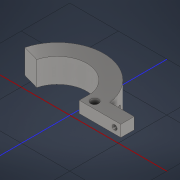
# Autodesk Inventor part: holder2_clamp
Saved by Autodesk Inventor 2021 (Build 250183000, 183)
## iProperties
Created: 2021-06-04
Part Number: holder2_clamp
Material: Steel, Mild
Document SubType Name: Modeling
Designer: Watchdog
Density: 7.85 g/cm^3
Appearance: Semi-Polished
Author: Watchdog
Autodesk Inventor part; units mm, degrees
ref_plane "YZ Plane" through (0, 0, 0) normal (1, 0, 0) x (0, 1, 0)
ref_plane "XZ Plane" through (0, 0, 0) normal (0, 1, 0) x (-1, 0, 0)
sketch "Sketch1" plane through (0, 0, 0) normal (0, 1, 0) x (-1, 0, 0)
  line L0 (5, 0) -> (16.619, -3)
  line L1 (5, 0) -> (-7, 0)
  arc A0 (-7, 0) -> (16.619, -3) centre (5, 0) ccw
  line L2 (0, 0) -> (-12, 0)
  arc A1 (-14, 0) -> (23.3548, -4.9094) centre (5, 0) ccw
  line L3 (16.619, -3) -> (23.3548, -4.9094)
  line L4 (-7, 0) -> (-14, 0)
  point P0 (-7, 0)
  dimension "d0" = 12
  dimension "d2" = 3
  dimension "d3" = 12
  dimension "d4" = 0
  dimension "d5" = 5
  dimension "d6" = 0
  dimension "d7" = 7
  constraints: 11 end point, 6 point on circle, 2 centre point, 2 horizontal, 1 coincident
  measures "d0" distance of L0.start L0.end
  measures "d2" vertical distance of L2.start L0.end
  measures "d3" distance of L2.start L2.end
  measures "d4" vertical distance of L2.start L0.start
  measures "d5" distance of L2.start L0.start
  measures "d6" distance between parallel lines of L2 L1
  measures "d7" radial gap between concentric circles of A1 A0
extrude "Extrusion1" add sketch "Sketch1" along normal blind 10 contours L3 A1 L4 L2 A0
ref_plane "Work Plane1" through (7, 0, -2.75) normal (0, 0, 1) x (1, 0, 0)
split "Split1" plane through (7, 0, -2.75) removes the side toward (0, 0, 1)
sketch "Sketch2" plane through (6.6806, 0, -2.75) normal (0, 0, 1) x (1, 0, 0)
  line L0 (0, 0) -> (0, 10) projected
  line L1 (7.1193, 0) -> (0, 0) projected
  line L2 (7.1193, 10) -> (7.1193, 0) projected
  line L3 (0, 10) -> (7.1193, 10) projected
  point P0 (-6.6806, 0)
extrude "Extrusion2" add sketch "Sketch2" along normal blind 5.5
sketch "Sketch3" plane through (13.7999, 0, -2.75) normal (1, 0, 0) x (0, 0, -1)
  line L0 (0, 10) -> (0, 0) projected
  line L1 (0, 10) -> (-5.5, 10) projected
  line L2 (-5.5, 0) -> (-5.5, 10) projected
  line L3 (0, 0) -> (-5.5, 0) projected
  point P0 (-2.75, 0)
extrude "Extrusion3" add sketch "Sketch3" along normal blind 10
sketch "Sketch4" plane through (0, 0, 0) normal (0, -1, 0) x (1, 0, 0)
  line L0 (6.6806, -2.75) -> (6.6806, 2.75) projected
  point P0 (0, 0)
  point P1 (10.2403, 0)
  point P2 (13.7999, -2.75)
  dimension "d15" = 0
  dimension "d16" = 3.5596
  dimension "d17" = 7.1193
  measures "d15" vertical distance of point (0, 0) point (10.24, 0)
  measures "d16" distance from line of L0 point (10.24, 0)
  measures "d17" distance of L0.start point (13.8, -2.75)
hole "Hole1" at (10.2403, 0, 0) direction (0, 1, 0) diameter 3.25 end through all
sketch "Sketch5" plane through (6.6806, 0, -2.75) normal (-1, 0, 0) x (0, 0, 1)
  line L0 (5.5, 0) -> (-6.5, 0)
  line L1 (-6.5, 0) -> (-6.5, 5.25)
  line L2 (-6.5, 5.25) -> (5.5, 5.25)
  line L3 (5.5, 5.25) -> (5.5, 0)
  line L4 (0, 12) -> (0, -2) projected
  dimension "d29" = 5.25
  dimension "d30" = 6.5
  constraints: 8 end point, 2 parallel, 1 horizontal, 1 perpendicular
  measures "d29" distance between parallel lines of L0 L2
  measures "d30" distance between parallel lines of L4 L1
extrude "halfCut" cut sketch "Sketch5" along normal blind 5.5 and the other way blind 20
fillet "Fillet1" radius 1 1 edges at (7.1204, 5.25, -9.25)
sketch "Sketch6" plane through (6.6806, 0, 2.75) normal (0, 0, 1) x (1, 0, 0)
  line L0 (0, 10) -> (17.1193, 10) projected
  line L1 (0, 5.25) -> (17.1193, 5.25) projected
  line L2 (17.1193, 10) -> (17.1193, 5.25) projected
  point P0 (-6.6806, 0)
  point P1 (14.6193, 7.625)
  dimension "d33" = 2.375
  dimension "d34" = 4.75
  dimension "d35" = 2.5
  measures "d33" distance from line of L0 point (14.619, 7.625)
  measures "d34" distance between parallel lines of L0 L1
  measures "d35" distance from line of L2 point (14.619, 7.625)
hole "Hole2" at (21.2999, 7.625, 2.75) direction (0, 0, -1) diameter 2 end through all
equation "\"d0\" = r"
equation "\"d2\" = 0.5 * a1"
equation "\"d3\" = r"
equation "\"d7\" = t"
equation "\"d11\" = a2"
equation "\"d16\" = 0.5 * d17"
equation "\"d18\" = dpin"
equation "\"d28\" = fillet"
equation "\"d33\" = 0.5 * d34"
equation "\"d36\" = dcable"
equation "\"r\" = 12"
equation "\"t\" = 7"
equation "\"a1\" = 6"
equation "\"a2\" = 5.5"
equation "\"d10\" = -0.5 * a2"
equation "\"dpin\" = 3.25"
equation "\"fillet\" = 1"
equation "\"dcable\" = 2"
body "Solid1"
